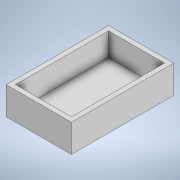
# Autodesk Inventor part: carcasa inferior
Saved by Autodesk Inventor 2020 (Build 240168000, 168)
## iProperties
Created: 2022-05-20
Part Number: carcasa inferior
Material: Generic
Document SubType Name: Modeling
Designer: juanc
Density: 1 g/cm^3
Appearance: Default
Author: juanc
Autodesk Inventor part; units mm, degrees
ref_plane "YZ Plane" through (0, 0, 0) normal (1, 0, 0) x (0, 1, 0)
ref_plane "XZ Plane" through (0, 0, 0) normal (0, 1, 0) x (-1, 0, 0)
ref_plane "XY Plane" through (0, 0, 0) normal (0, 0, 1) x (1, 0, 0)
sketch "Sketch1" plane through (0, 0, 0) normal (0, 1, 0) x (-1, 0, 0)
  line L0 (0, 0) -> (60, 0)
  line L1 (60, 0) -> (60, -100)
  line L2 (60, -100) -> (0, -100)
  line L3 (0, -100) -> (0, 0)
  line L4 (60, 0) -> (0, -100) construction
  line L5 (60, -100) -> (0, 0) construction
  line L6 (-5, 5) -> (65, 5)
  line L7 (65, 5) -> (65, -105)
  line L8 (65, -105) -> (-5, -105)
  line L9 (-5, -105) -> (-5, 5)
  line L10 (-5, 5) -> (65, -105) construction
  line L11 (65, 5) -> (-5, -105) construction
  point P0 (30, -50)
  dimension "d0" = 60
  dimension "d1" = 100
  dimension "d2" = 70
  dimension "d3" = 110
  constraints: 24 end point, 4 parallel, 3 midpoint, 2 horizontal, 2 perpendicular
  measures "d0" distance of L1.end L2.end
  measures "d1" distance of L0.end L1.end
  measures "d2" distance of L7.end L8.end
  measures "d3" distance of L6.end L7.end
extrude "Extrusion1" add sketch "Sketch1" along normal blind 30
extrude "Extrusion2" add sketch "Sketch1" along normal blind 5 contours L0 L1 L2 L3
body "Solid1"
